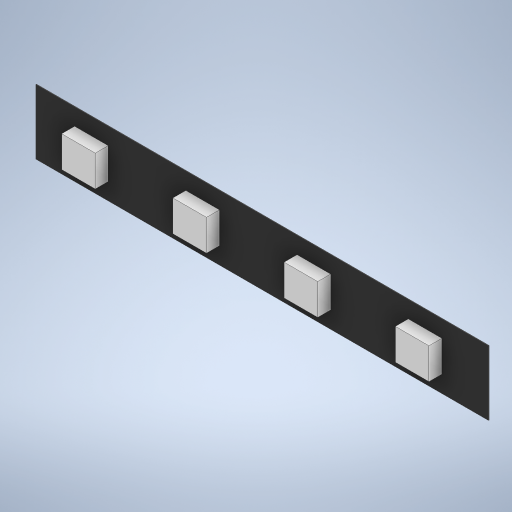
# Autodesk Inventor part: 네오픽셀
Saved by Autodesk Inventor 2023 (Build 270158000, 158)
## iProperties
Created: 2022-11-10
Part Number: 네오픽셀
Material: 일반
Document SubType Name: Modeling
Designer: user
Density: 1 g/cm^3
Appearance: 기본값
Author: user
Autodesk Inventor part; units mm, degrees
ref_plane "YZ Plane" through (0, 0, 0) normal (1, 0, 0) x (0, 1, 0)
ref_plane "XZ Plane" through (0, 0, 0) normal (0, 1, 0) x (-1, 0, 0)
ref_plane "XY Plane" through (0, 0, 0) normal (0, 0, 1) x (1, 0, 0)
sketch "스케치1" plane through (0, 0, 0) normal (0, 0, 1) x (1, 0, 0)
  line L0 (-35, 5) -> (35, 5)
  line L1 (35, 5) -> (35, -5)
  line L2 (35, -5) -> (-35, -5)
  line L3 (-35, -5) -> (-35, 5)
  line L4 (-35, 5) -> (35, -5) construction
  line L5 (35, 5) -> (-35, -5) construction
  point P0 (0, 0)
  dimension "d0" = 70
  dimension "d1" = 10
  constraints: 12 end point, 2 midpoint, 2 parallel, 1 horizontal, 1 perpendicular
  measures "d0" distance of L1.end L2.end
  measures "d1" distance of L0.end L1.end
extrude "돌출1" add sketch "스케치1" along normal blind 0.1
sketch "스케치2" plane through (0, 0, 0.1) normal (0, 0, 1) x (1, 0, 0)
  line L0 (-29, -2.4) -> (-23.8, -2.4)
  line L1 (-23.8, -2.4) -> (-23.8, 2.4)
  line L2 (-23.8, 2.4) -> (-29, 2.4)
  line L3 (-29, 2.4) -> (-29, -2.4)
  line L4 (-29, -2.4) -> (-23.8, 2.4) construction
  line L5 (-23.8, -2.4) -> (-29, 2.4) construction
  line L6 (-35, 5) -> (-35, -5) projected
  line L7 (-11.8, -2.4) -> (-6.6, -2.4)
  line L8 (-6.6, -2.4) -> (-6.6, 2.4)
  line L9 (-6.6, 2.4) -> (-11.8, 2.4)
  line L10 (-11.8, 2.4) -> (-11.8, -2.4)
  line L11 (-11.8, -2.4) -> (-6.6, 2.4) construction
  line L12 (-6.6, -2.4) -> (-11.8, 2.4) construction
  line L13 (5.4, -2.4) -> (10.6, -2.4)
  line L14 (10.6, -2.4) -> (10.6, 2.4)
  line L15 (10.6, 2.4) -> (5.4, 2.4)
  line L16 (5.4, 2.4) -> (5.4, -2.4)
  line L17 (5.4, -2.4) -> (10.6, 2.4) construction
  line L18 (10.6, -2.4) -> (5.4, 2.4) construction
  line L19 (22.6, -2.4) -> (27.8, -2.4)
  line L20 (27.8, -2.4) -> (27.8, 2.4)
  line L21 (27.8, 2.4) -> (22.6, 2.4)
  line L22 (22.6, 2.4) -> (22.6, -2.4)
  line L23 (22.6, -2.4) -> (27.8, 2.4) construction
  line L24 (27.8, -2.4) -> (22.6, 2.4) construction
  point P0 (0, 0)
  point P1 (-26.4, 0)
  point P2 (-9.2, 0)
  point P3 (8, 0)
  point P4 (25.2, 0)
  dimension "d4" = 5.2
  dimension "d5" = 4.8
  dimension "d6" = 6
  dimension "d9" = 17.2
  constraints: 48 end point, 2 horizontal, 2 midpoint, 2 parallel, 1 collinear, 1 horizontal alignment, 1 perpendicular, 32 other
  measures "d4" distance of L2.end L1.end
  measures "d5" distance of L1.end L0.end
  measures "d6" distance between parallel lines of L6 L3
  measures "d9" distance of L0.start L7.start
extrude "돌출2" add sketch "스케치2" along normal blind 2
